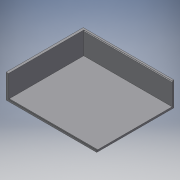
# Autodesk Inventor part: Batcap2
Saved by Autodesk Inventor 2016 SP2 (Build 200236200, 236)
## iProperties
Created: 2018-06-26
Part Number: Batcap2
Material: Generisch
Document SubType Name: Modeling
Designer: Nils
Density: 1 g/cm^3
Appearance: Vorgabe
Author: Nils
Autodesk Inventor part; units mm, degrees
ref_plane "YZ Plane" through (0, 0, 0) normal (1, 0, 0) x (0, 1, 0)
ref_plane "XZ Plane" through (0, 0, 0) normal (0, 1, 0) x (-1, 0, 0)
ref_plane "XY Plane" through (0, 0, 0) normal (0, 0, 1) x (1, 0, 0)
sketch "Skizze1" plane through (0, 0, 0) normal (1, 0, 0) x (0, 1, 0)
  line L0 (123.2117, 108.1983) -> (122.2117, 109.1983) construction
  line L1 (122.2117, 133.1983) -> (122.2117, 107.1983) construction
  line L2 (122.2117, 107.1983) -> (205.2117, 107.1983) construction
  line L3 (205.2117, 107.1983) -> (205.2117, 133.1983) construction
  line L4 (203.2117, 133.1983) -> (204.2117, 132.1983) construction
  line L5 (122.2117, 107.1983) -> (205.2117, 107.1983)
  line L6 (205.2117, 107.1983) -> (205.2117, 133.1983)
  line L7 (203.2117, 109.1983) -> (123.2703, 109.1983)
  line L8 (123.1703, 108.0983) -> (122.2117, 109.0569)
  line L9 (122.2117, 109.0569) -> (122.2117, 107.1983)
  line L10 (123.2703, 108.0983) -> (123.2703, 109.1983)
  line L11 (123.1703, 108.0983) -> (123.2703, 108.0983)
  line L12 (203.3531, 133.1983) -> (204.3531, 132.1983)
  line L13 (205.2117, 133.1983) -> (203.3531, 133.1983)
  line L14 (204.3531, 132.1983) -> (204.3531, 132.0483)
  line L15 (204.3531, 132.0483) -> (203.2117, 132.0483)
  line L16 (203.2117, 132.0483) -> (203.2117, 109.1983)
  point P0 (0, 0)
  dimension "d2" = 0.1
  dimension "d4" = 2
  dimension "d6" = 1.1
  dimension "d8" = 0.1
  dimension "d9" = 0.1
  dimension "d10" = 0.15
  dimension "d11" = 2
  constraints: 25 end point, 3 parallel, 3 perpendicular, 2 collinear, 2 horizontal, 2 vertical, 1 point on line
  measures "d2" distance between parallel lines of L8 L0
  measures "d4" distance between parallel lines of L7 L2
  measures "d6" distance of L10.start L7.end
  measures "d8" distance of L8.start L10.start
  measures "d9" distance between parallel lines of L4 L12
  measures "d10" distance of L12.end L14.end
  measures "d11" distance between parallel lines of L3 L16
extrude "Extrusion1" add sketch "Skizze1" along normal blind 95
sketch "Skizze2" plane through (0, 0, 0) normal (-1, 0, 0) x (0, 0, 1)
  line L0 (107.1983, 205.2117) -> (133.1983, 205.2117) projected
  line L1 (109.0569, 122.2117) -> (107.1983, 122.2117) projected
  line L2 (133.1983, 205.2117) -> (107.1983, 205.2117)
  line L3 (107.1983, 205.2117) -> (107.1983, 122.2117)
  line L4 (107.1983, 122.2117) -> (133.1983, 122.2117)
  line L5 (133.1983, 122.2117) -> (133.1983, 205.2117)
  point P0 (0, 0)
  constraints: 8 end point, 2 parallel, 1 horizontal, 1 perpendicular
extrude "Extrusion2" add sketch "Skizze2" along normal blind 2.5
